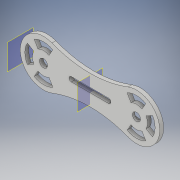
# Autodesk Inventor part: pierna1_2
Saved by Autodesk Inventor 2019 (Build 230136000, 136)
## iProperties
Created: 2020-02-11
Part Number: pierna1_2
Material: Generic
Document SubType Name: Modeling
Designer: jacqu
Density: 1 g/cm^3
Appearance: Default
d0: 20.000 mm
Author: jacqu
Autodesk Inventor part; units mm, degrees
ref_plane "YZ Plane" through (0, 0, 0) normal (1, 0, 0) x (0, 1, 0)
ref_plane "XZ Plane" through (0, 0, 0) normal (0, 1, 0) x (-1, 0, 0)
ref_plane "XY Plane" through (0, 0, 0) normal (0, 0, 1) x (1, 0, 0)
sketch "Sketch1" plane through (0, 0, 0) normal (0, 0, 1) x (1, 0, 0)
  arc A0 (-72.7273, 18.6308) -> (-72.7273, -18.6308) centre (-80, 0) ccw
  arc A1 (-7.2727, -18.6308) -> (-72.7273, -18.6308) centre (-40, -102.4695) ccw
  arc A2 (-7.2727, -18.6308) -> (-7.2727, 18.6308) centre (0, 0) ccw
  arc A3 (-72.7273, 18.6308) -> (-7.2727, 18.6308) centre (-40, 102.4695) ccw
  line L0 (-79.6316, -3.4604) -> (-65.8083, -1.9888)
  arc A4 (-79.6316, 3.4604) -> (-79.6316, -3.4604) centre (-80, 0) ccw
  line L1 (-79.6316, 3.4604) -> (-65.8083, 1.9888)
  arc A5 (-65.8083, -1.9888) -> (-65.8083, 1.9888) centre (-66.02, 0) ccw
  line L2 (-0.3684, -3.4604) -> (-14.1917, -1.9888)
  arc A6 (-14.1917, 1.9888) -> (-14.1917, -1.9888) centre (-13.98, 0) ccw
  line L3 (-0.3684, 3.4604) -> (-14.1917, 1.9888)
  arc A7 (-0.3684, -3.4604) -> (-0.3684, 3.4604) centre (0, 0) ccw
  arc A8 (-80.3684, -3.4604) -> (-80.3684, 3.4604) centre (-80, 0) ccw
  point P0 (-103.8261, -115.9088)
  dimension "d0" = 20
  dimension "d1" = 20
  dimension "d2" = 90
  dimension "d3" = 90
  dimension "d4" = 3.48
  dimension "d6" = 2
  dimension "d7" = 80
  dimension "d11" = 19.46
  dimension "d33" = 3.48
  constraints: 20 point on circle, 11 tangent, 9 centre point, 8 end point, 3 coincident, 3 equal length, 3 horizontal alignment, 2 equal radius
  measures "d0" radius of A0
  measures "d1" radius of A2
  measures "d2" radius of A3
  measures "d3" radius of A1
  measures "d4" radius of A4
  measures "d6" radius of A5
  measures "d7" distance of A7.centre A4.centre
  measures "d33" radius of A8
extrude "Extrusion1" add sketch "Sketch1" along normal blind 3.3
sketch "Sketch3" plane through (0, 0, 3.3) normal (0, 0, 1) x (1, 0, 0)
  arc A0 (-14.1917, 1.9888) -> (-14.1917, -1.9888) centre (-13.98, 0) ccw projected
  line L0 (-14.1917, 1.9888) -> (-0.3684, 3.4604) projected
  arc A1 (-0.3684, -3.4604) -> (-0.3684, 3.4604) centre (0, 0) ccw projected
  line L1 (-0.3684, -3.4604) -> (-14.1917, -1.9888) projected
  arc A2 (-79.6316, 3.4604) -> (-79.6316, -3.4604) centre (-80, 0) ccw projected
  line L2 (-79.6316, 3.4604) -> (-65.8083, 1.9888) projected
  arc A3 (-65.8083, -1.9888) -> (-65.8083, 1.9888) centre (-66.02, 0) ccw projected
  line L3 (-65.8083, -1.9888) -> (-79.6316, -3.4604) projected
  arc A4 (-72.7273, 18.6308) -> (-72.7273, -18.6308) centre (-80, 0) ccw projected
  arc A5 (-7.2727, -18.6308) -> (-72.7273, -18.6308) centre (-40, -102.4695) ccw projected
  arc A6 (-7.2727, -18.6308) -> (-7.2727, 18.6308) centre (0, 0) ccw projected
  arc A7 (-72.7273, 18.6308) -> (-7.2727, 18.6308) centre (-40, 102.4695) ccw projected
  line L4 (-56.02, 2) -> (-23.98, 2)
  line L5 (-56.02, -2) -> (-23.98, -2)
  arc A8 (-56.02, 2) -> (-56.02, -2) centre (-56.02, 0) ccw
  arc A9 (-23.98, -2) -> (-23.98, 2) centre (-23.98, 0) ccw
  point P0 (-83.48, 0)
  dimension "d12" = 2
  dimension "d13" = 10
  dimension "d14" = 10
  constraints: 5 point on circle, 4 end point, 4 tangent, 2 centre point, 2 horizontal, 1 horizontal alignment
  measures "d12" radius of A8
  measures "d13" distance of A3.centre A8.centre
  measures "d14" distance of A0.centre A9.centre
extrude "Extrusion2" cut sketch "Sketch3" against normal blind 3.3 contours L4 A9 L5 A8
sketch "Sketch5" plane through (0, 0, 3.3) normal (0, 0, 1) x (1, 0, 0)
  arc A0 (-56.02, 2) -> (-56.02, -2) centre (-56.02, 0) ccw projected
  line L0 (-56.02, 2) -> (-23.98, 2) projected
  arc A1 (-23.98, -2) -> (-23.98, 2) centre (-23.98, 0) ccw projected
  line L1 (-23.98, -2) -> (-56.02, -2) projected
  arc A2 (-14.1917, 1.9888) -> (-14.1917, -1.9888) centre (-13.98, 0) ccw projected
  line L2 (-14.1917, 1.9888) -> (-0.3684, 3.4604) projected
  arc A3 (-0.3684, -3.4604) -> (-0.3684, 3.4604) centre (0, 0) ccw projected
  line L3 (-0.3684, -3.4604) -> (-14.1917, -1.9888) projected
  arc A4 (-79.6316, 3.4604) -> (-79.6316, -3.4604) centre (-80, 0) ccw projected
  line L4 (-79.6316, 3.4604) -> (-65.8083, 1.9888) projected
  arc A5 (-65.8083, -1.9888) -> (-65.8083, 1.9888) centre (-66.02, 0) ccw projected
  line L5 (-65.8083, -1.9888) -> (-79.6316, -3.4604) projected
  arc A6 (-72.7273, 18.6308) -> (-72.7273, -18.6308) centre (-80, 0) ccw projected
  arc A7 (-7.2727, -18.6308) -> (-72.7273, -18.6308) centre (-40, -102.4695) ccw projected
  arc A8 (-7.2727, -18.6308) -> (-7.2727, 18.6308) centre (0, 0) ccw projected
  arc A9 (-72.7273, 18.6308) -> (-7.2727, 18.6308) centre (-40, 102.4695) ccw projected
  circle A10 centre (-80, 0) radius 9.48 construction
  circle A11 centre (-80, 0) radius 16 construction
  line L6 (-80, 0) -> (-88, 13.8564) construction
  line L7 (-80, 0) -> (-72, 13.8564) construction
  line L8 (-80, 0) -> (-88, -13.8564) construction
  line L9 (-80, 0) -> (-72, -13.8564) construction
  line L10 (-80, 0) -> (-93.8564, -8) construction
  line L11 (-80, 0) -> (-93.8564, 8) construction
  line L12 (-80, 0) -> (-66.02, 0) construction
  arc A12 (-88.2099, 4.74) -> (-88.2099, -4.74) centre (-80, 0) ccw
  arc A13 (-93.8564, 8) -> (-93.8564, -8) centre (-80, 0) ccw
  arc A14 (-75.26, 8.2099) -> (-84.74, 8.2099) centre (-80, 0) ccw
  arc A15 (-84.74, -8.2099) -> (-75.26, -8.2099) centre (-80, 0) ccw
  line L13 (-93.8564, -8) -> (-88.2099, -4.74)
  line L14 (-93.8564, 8) -> (-88.2099, 4.74)
  line L15 (-88, 13.8564) -> (-84.74, 8.2099)
  line L16 (-75.26, 8.2099) -> (-72, 13.8564)
  line L17 (-84.74, -8.2099) -> (-88, -13.8564)
  line L18 (-75.26, -8.2099) -> (-72, -13.8564)
  arc A16 (-88, -13.8564) -> (-72, -13.8564) centre (-80, 0) ccw
  arc A17 (-72, 13.8564) -> (-88, 13.8564) centre (-80, 0) ccw
  dimension "d20" = 60
  dimension "d21" = 60
  dimension "d23" = 60
  dimension "d24" = 30
  dimension "d26" = 20
  dimension "d27" = 32
  dimension "d28" = 18.96
  dimension "d29" = 3.48
  constraints: 26 end point, 25 point on circle, 8 centre point, 8 concentric, 8 point on line, 7 collinear, 2 coincident, 1 horizontal
  measures "d20" angle of L7 L6
  measures "d21" angle of L10 L11
  measures "d23" angle of L12 L7
  measures "d24" angle of L6 L11
  measures "d26" radius of A6
  measures "d27" diameter of A11
  measures "d28" diameter of A10
  measures "d29" radius of A4
extrude "Extrusion3" cut sketch "Sketch5" against normal blind 3.3 contours A12 L13 A13 L14 | A14 L15 A17 L16 | A15 L18 A16 L17
ref_plane "Work Plane2" through (-40, 0, 3.3) normal (-1, 0, 0) x (0, -1, 0)
ref_plane "Work Plane1" through (-100, 0, 3.3) normal (-1, 0, 0) x (0, -1, 0)
mirror "Mirror1" about plane through (-40, 0, 3.3) normal (-1, 0, 0) of "Extrusion3"
sketch "Sketch6" plane through (0, 0, 3.3) normal (0, 0, 1) x (1, 0, 0)
  arc A0 (4.74, 8.2099) -> (-4.74, 8.2099) centre (0, 0) ccw projected
  line L0 (-4.74, 8.2099) -> (-8, 13.8564) projected
  arc A1 (8, 13.8564) -> (-8, 13.8564) centre (0, 0) ccw projected
  line L1 (8, 13.8564) -> (4.74, 8.2099) projected
  line L2 (13.8564, -8) -> (8.2099, -4.74) projected
  arc A2 (8.2099, -4.74) -> (8.2099, 4.74) centre (0, 0) ccw projected
  line L3 (8.2099, 4.74) -> (13.8564, 8) projected
  arc A3 (13.8564, -8) -> (13.8564, 8) centre (0, 0) ccw projected
  arc A4 (-4.74, -8.2099) -> (4.74, -8.2099) centre (0, 0) ccw projected
  line L4 (4.74, -8.2099) -> (8, -13.8564) projected
  arc A5 (-8, -13.8564) -> (8, -13.8564) centre (0, 0) ccw projected
  line L5 (-8, -13.8564) -> (-4.74, -8.2099) projected
  arc A6 (-75.26, 8.2099) -> (-84.74, 8.2099) centre (-80, 0) ccw projected
  line L6 (-84.74, 8.2099) -> (-88, 13.8564) projected
  arc A7 (-72, 13.8564) -> (-88, 13.8564) centre (-80, 0) ccw projected
  line L7 (-72, 13.8564) -> (-75.26, 8.2099) projected
  line L8 (-88.2099, -4.74) -> (-93.8564, -8) projected
  arc A8 (-93.8564, 8) -> (-93.8564, -8) centre (-80, 0) ccw projected
  line L9 (-93.8564, 8) -> (-88.2099, 4.74) projected
  arc A9 (-88.2099, 4.74) -> (-88.2099, -4.74) centre (-80, 0) ccw projected
  arc A10 (-84.74, -8.2099) -> (-75.26, -8.2099) centre (-80, 0) ccw projected
  line L10 (-75.26, -8.2099) -> (-72, -13.8564) projected
  arc A11 (-88, -13.8564) -> (-72, -13.8564) centre (-80, 0) ccw projected
  line L11 (-88, -13.8564) -> (-84.74, -8.2099) projected
  arc A12 (-56.02, 2) -> (-56.02, -2) centre (-56.02, 0) ccw projected
  line L12 (-56.02, 2) -> (-23.98, 2) projected
  arc A13 (-23.98, -2) -> (-23.98, 2) centre (-23.98, 0) ccw projected
  line L13 (-23.98, -2) -> (-56.02, -2) projected
  arc A14 (-14.1917, 1.9888) -> (-14.1917, -1.9888) centre (-13.98, 0) ccw projected
  line L14 (-14.1917, 1.9888) -> (-0.3684, 3.4604) projected
  arc A15 (-0.3684, -3.4604) -> (-0.3684, 3.4604) centre (0, 0) ccw projected
  line L15 (-0.3684, -3.4604) -> (-14.1917, -1.9888) projected
  arc A16 (-79.6316, 3.4604) -> (-79.6316, -3.4604) centre (-80, 0) ccw projected
  line L16 (-79.6316, 3.4604) -> (-65.8083, 1.9888) projected
  arc A17 (-65.8083, -1.9888) -> (-65.8083, 1.9888) centre (-66.02, 0) ccw projected
  line L17 (-65.8083, -1.9888) -> (-79.6316, -3.4604) projected
  arc A18 (-72.7273, 18.6308) -> (-72.7273, -18.6308) centre (-80, 0) ccw projected
  arc A19 (-7.2727, -18.6308) -> (-72.7273, -18.6308) centre (-40, -102.4695) ccw projected
  arc A20 (-7.2727, -18.6308) -> (-7.2727, 18.6308) centre (0, 0) ccw projected
  arc A21 (-72.7273, 18.6308) -> (-7.2727, 18.6308) centre (-40, 102.4695) ccw projected
  arc A22 (-79.6316, 3.4604) -> (-79.6316, -3.4604) centre (-80, 0) ccw projected
  line L18 (-65.8083, -1.9888) -> (-79.6316, -3.4604) projected
  arc A23 (-65.8083, -1.9888) -> (-65.8083, 1.9888) centre (-66.02, 0) ccw
  arc A24 (-65.8083, -1.9888) -> (-65.8083, 1.9888) centre (-66.02, 0) ccw projected
  line L19 (-79.6316, -3.4604) -> (-65.8083, -1.9888)
  line L20 (-79.6316, 3.4604) -> (-65.8083, 1.9888) projected
  arc A25 (-79.6316, -3.4604) -> (-79.6316, 3.4604) centre (-80, 0) ccw
  line L21 (-79.6316, 3.4604) -> (-65.8083, 1.9888)
  constraints: 5 tangent, 4 end point, 4 point on circle, 2 centre point, 1 collinear, 1 concentric
extrude "Extrusion4" add sketch "Sketch6" against normal blind 2 contours L16 A17 L17 A25
mirror "Mirror2" about plane through (-40, 0, 3.3) normal (-1, 0, 0) of "Extrusion4"
equation "\"d0\" = radio_muslo"
equation "\"d1\" = d0"
equation "\"d2\" = curva"
equation "\"d3\" = d2"
equation "\"d7\" = distancia_centros"
equation "\"d33\" = d4"
equation "\"d8\" = espesor"
equation "\"curva\" = 90"
equation "\"distancia_centros\" = 80"
equation "\"espesor\" = 3.3"
equation "\"radio_muslo\" = 20"
body "Solid1"
